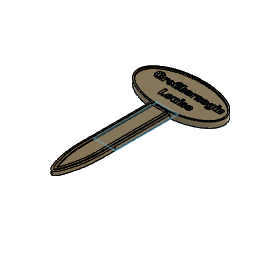
Rosen-Tafel_Großherzoging_Louise v2 (Autodesk Fusion 360 design; units mm, degrees)
Autodesk Fusion 360 part; units mm, degrees
(part 1 of 2)
sketch "Skizze1" plane through (0, 0, 0) normal (0, 0, 1) x (1, 0, 0) in component "Tafe"
  ellipse E0 centre (0, 0) end of major axis (60, 0) minor radius 30
  line L0 (-60, 0) -> (60, 0)
  line L1 (0, -30) -> (0, 30)
  dimension "d1" = 60
  constraint coincident E0.centre origin
  constraint horizontal L0
  constraint coincident E0 L0.start
  constraint coincident E0 L0.end
  constraint coincident E0 L1.start
  constraint coincident E0 L1.end
  measures "d1" distance of E0
extrude "Extrusion1" add sketch "Skizze1" along normal blind 3 makes body 1 in component "Tafe"
sketch "Skizze2" plane through (0, 0, 3) normal (0, 0, 1) x (-1, 0, 0) in component "Tafe"
  ellipse E0 centre (0, 0) end of major axis (-60, 0) minor radius 30
  spline S0 degree 3 poles (61.9509, 0) (61.9509, 4.2635) (60.3055, 8.4828) (57.3091, 12.2636) (52.6449, 18.1488) (44.7166, 23.0684) (34.8255, 26.4973) (25.2136, 29.8294) (13.7584, 31.7256) (2.1658, 31.9316) (-9.8896, 32.1459) (-22.0459, 30.5274) (-32.3487, 27.3124) (-41.3637, 24.4992) (-48.9522, 20.4892) (-54.1681, 15.6411) (-58.1005, 11.9859) (-60.7028, 7.8251) (-61.5993, 3.4465) (-62.4053, -0.4903) (-61.7899, -4.5541) (-59.8722, -8.3093) (-56.3973, -15.1137) (-48.7697, -20.9418) (-38.5998, -25.0786) (-29.6788, -28.7075) (-18.796, -31.0188) (-7.5068, -31.7189) (4.0223, -32.434) (15.9353, -31.462) (26.4461, -28.9362) (36.7725, -26.4548) (45.7187, -22.4959) (52.0049, -17.4981) (56.4978, -13.926) (59.6597, -9.8063) (61.0885, -5.3839) (61.6588, -3.6187) (61.9509, -1.8099) (61.9509, 0) knots -3.141593 -3.141593 -3.141593 -3.141593 -2.764311 -2.764311 -2.764311 -2.177028 -2.177028 -2.177028 -1.606323 -1.606323 -1.606323 -1.012833 -1.012833 -1.012833 -0.49353 -0.49353 -0.49353 -0.102016 -0.102016 -0.102016 0.249996 0.249996 0.249996 0.887852 0.887852 0.887852 1.447382 1.447382 1.447382 2.018805 2.018805 2.018805 2.580199 2.580199 2.580199 2.981436 2.981436 2.981436 3.141593 3.141593 3.141593 3.141593
  dimension "d4" = 1.9509
extrude "Extrusion2" add sketch "Skizze2" along normal blind 2 and the other way blind 2 bodies 1 in component "Tafe"
sketch "Skizze3" plane through (0, 0, 0) normal (0, 0, 1) x (1, 0, 0) in component "Tafe"
extrude "Extrusion3" add 1 faces at (23.0091, -28.1834, 1) along direction (0, 0, -1) blind 1 on bodies 1 bodies 1 in component "Tafe"
sketch "Skizze1 (2)" plane through (0, 0, 0) normal (0, 0, 1) x (1, 0, 0) in component "Ständer"
extrude "Extrusion4" add 2 faces at (23.0091, -28.1834, 0) (8.4972, -9.7981, 0) along direction (0, 0, -1) blind 3 on bodies 1 bodies 1 in component "Tafe"
sketch "Skizze2 (2)" plane through (0, 0, -3) normal (0, 0, -1) x (1, 0, 0) in component "Ständer"
  spline S0 degree 3 poles (-61.9509, 0) (-61.9509, -1.8099) (-61.6588, -3.6187) (-61.0885, -5.3839) (-59.6597, -9.8063) (-56.4978, -13.926) (-52.0049, -17.4981) (-45.7187, -22.4959) (-36.7725, -26.4548) (-26.4461, -28.9362) (-15.9353, -31.462) (-4.0223, -32.434) (7.5068, -31.7189) (18.796, -31.0188) (29.6788, -28.7075) (38.5998, -25.0786) (48.7697, -20.9418) (56.3973, -15.1137) (59.8722, -8.3093) (61.7899, -4.5541) (62.4053, -0.4903) (61.5993, 3.4465) (60.7028, 7.8251) (58.1005, 11.9859) (54.1681, 15.6411) (48.9522, 20.4892) (41.3637, 24.4992) (32.3487, 27.3124) (22.0459, 30.5274) (9.8896, 32.1459) (-2.1658, 31.9316) (-13.7584, 31.7256) (-25.2136, 29.8294) (-34.8255, 26.4973) (-44.7166, 23.0684) (-52.6449, 18.1488) (-57.3091, 12.2636) (-60.3055, 8.4828) (-61.9509, 4.2635) (-61.9509, 0) knots -3.141593 -3.141593 -3.141593 -3.141593 -2.981436 -2.981436 -2.981436 -2.580199 -2.580199 -2.580199 -2.018805 -2.018805 -2.018805 -1.447382 -1.447382 -1.447382 -0.887852 -0.887852 -0.887852 -0.249996 -0.249996 -0.249996 0.102016 0.102016 0.102016 0.49353 0.49353 0.49353 1.012833 1.012833 1.012833 1.606323 1.606323 1.606323 2.177028 2.177028 2.177028 2.764311 2.764311 2.764311 3.141593 3.141593 3.141593 3.141593
  line L0 (15, 20) -> (-15, 20)
  line L1 (-15, 20) -> (-15, 110)
  line L2 (-15, 110) -> (15, 110)
  line L3 (15, 110) -> (15, 20)
  constraint horizontal L0
  constraint vertical L1
  constraint horizontal L2
  constraint vertical L3
extrude "Extrusion1'" add sketch "Skizze2 (2)" against normal blind 5 separate body contours S0 L0 L1 L3 picked at (1.6815, 23.9477) makes body 2 in component "Ständer"
extrude "Extrusion2'" add sketch "Skizze2 (2)" against normal blind 5 contours S0 L1 L2 L3 bodies 2 in component "Ständer"
sketch "Skizze3 (2)" plane through (0, 0, 2) normal (0, 0, 1) x (-1, 0, 0) in component "Ständer"
  line L0 (15, 20) -> (15, 110)
  line L1 (15, 110) -> (-15, 110)
  line L2 (-15, 110) -> (-15, 20)
  line L3 (-15, 20) -> (15, 20)
  spline S0 degree 5 poles (15, 110) (15.0176, 110.8619) (15.0503, 112.5708) (15.0915, 115.0899) (15.1309, 118.3598) (15.1537, 122.2987) (15.1484, 126.0898) (15.1122, 129.7366) (15.0406, 133.2467) (14.9275, 136.6331) (14.7639, 139.9163) (14.5397, 143.1226) (14.2439, 146.2818) (13.867, 149.4242) (13.4012, 152.5784) (12.8426, 155.769) (12.1915, 159.0132) (11.4507, 162.3163) (10.6251, 165.6668) (9.72, 169.0317) (8.7408, 172.3517) (7.6913, 175.5347) (6.574, 178.4677) (5.3908, 181.0335) (4.1426, 183.1253) (2.8302, 184.6621) (1.7296, 185.4171) (0.8758, 185.7125) (0.294, 185.7893) (0, 185.7977) knots 0 0 0 0 0 0 0.04 0.08 0.12 0.16 0.2 0.24 0.28 0.32 0.36 0.4 0.44 0.48 0.52 0.56 0.6 0.64 0.68 0.72 0.76 0.8 0.84 0.88 0.92 0.96 1 1 1 1 1 1
  line L4 (0, -2.5) -> (0, -20)
  spline S1 degree 5 poles (-15, 110) (-15.0176, 110.8619) (-15.0503, 112.5708) (-15.0915, 115.0899) (-15.1309, 118.3598) (-15.1537, 122.2987) (-15.1484, 126.0898) (-15.1122, 129.7366) (-15.0406, 133.2467) (-14.9275, 136.6331) (-14.7639, 139.9163) (-14.5397, 143.1226) (-14.2439, 146.2818) (-13.867, 149.4242) (-13.4012, 152.5784) (-12.8426, 155.769) (-12.1915, 159.0132) (-11.4507, 162.3163) (-10.6251, 165.6668) (-9.72, 169.0317) (-8.7408, 172.3517) (-7.6913, 175.5347) (-6.574, 178.4677) (-5.3908, 181.0335) (-4.1426, 183.1253) (-2.8302, 184.6621) (-1.7296, 185.4171) (-0.8758, 185.7125) (-0.294, 185.7893) (0, 185.7977) knots 0 0 0 0 0 0 0.04 0.08 0.12 0.16 0.2 0.24 0.28 0.32 0.36 0.4 0.44 0.48 0.52 0.56 0.6 0.64 0.68 0.72 0.76 0.8 0.84 0.88 0.92 0.96 1 1 1 1 1 1
  line L5 (14.8117, 100.8471) -> (15.1883, 119.1529)
  line L6 (6.7737, 185.6047) -> (-6.7737, 185.9906)
  line L7 (-14.8117, 100.8471) -> (-15.1883, 119.1529)
  line L8 (-6.7737, 185.6047) -> (6.7737, 185.9906)
  point P0 (15, 134.2579)
  point P1 (13.5579, 151.4378)
  point P2 (9.54, 169.5876)
  point P3 (3.9981, 183.1652)
  point P4 (-15, 134.2579)
  point P5 (-13.5579, 151.4378)
  point P6 (-9.54, 169.5876)
  point P7 (-3.9981, 183.1652)
  constraint coincident L0.end L1.start
  constraint midpoint L0.end L5
  constraint midpoint S0.end L6
  constraint symmetric L0.end L4 L1.end
  constraint symmetric P0 L4 P4
  constraint symmetric P1 L4 P5
  constraint symmetric P2 L4 P6
  constraint symmetric P3 L4 P7
  constraint symmetric S0.end L4 S1.end
  constraint symmetric L4 L5.start L7.start
  constraint symmetric L4 L5.end L7.end
  constraint symmetric L4 L6.start L8.start
  constraint symmetric L4 L6.end L8.end
extrude "Extrusion3'" add sketch "Skizze3 (2)" against normal blind 5 contours L1 S0 S1 bodies 2 in component "Ständer"
sketch "Skizze4" plane through (0, 0, 2) normal (0, 0, 1) x (-1, 0, 0) in component "Ständer"
  line L0 (15, 20) -> (15, 110)
  spline S0 degree 5 poles (15, 110) (15.0176, 110.8619) (15.0503, 112.5708) (15.0915, 115.0899) (15.1309, 118.3598) (15.1537, 122.2987) (15.1484, 126.0898) (15.1122, 129.7366) (15.0406, 133.2467) (14.9275, 136.6331) (14.7639, 139.9163) (14.5397, 143.1226) (14.2439, 146.2818) (13.867, 149.4242) (13.4012, 152.5784) (12.8426, 155.769) (12.1915, 159.0132) (11.4507, 162.3163) (10.6251, 165.6668) (9.72, 169.0317) (8.7408, 172.3517) (7.6913, 175.5347) (6.574, 178.4677) (5.3908, 181.0335) (4.1426, 183.1253) (2.8302, 184.6621) (1.7296, 185.4171) (0.8758, 185.7125) (0.294, 185.7893) (0, 185.7977) knots 0 0 0 0 0 0 0.04 0.08 0.12 0.16 0.2 0.24 0.28 0.32 0.36 0.4 0.44 0.48 0.52 0.56 0.6 0.64 0.68 0.72 0.76 0.8 0.84 0.88 0.92 0.96 1 1 1 1 1 1
  spline S1 degree 5 poles (-15, 110) (-15.0176, 110.8619) (-15.0503, 112.5708) (-15.0915, 115.0899) (-15.1309, 118.3598) (-15.1537, 122.2987) (-15.1484, 126.0898) (-15.1122, 129.7366) (-15.0406, 133.2467) (-14.9275, 136.6331) (-14.7639, 139.9163) (-14.5397, 143.1226) (-14.2439, 146.2818) (-13.867, 149.4242) (-13.4012, 152.5784) (-12.8426, 155.769) (-12.1915, 159.0132) (-11.4507, 162.3163) (-10.6251, 165.6668) (-9.72, 169.0317) (-8.7408, 172.3517) (-7.6913, 175.5347) (-6.574, 178.4677) (-5.3908, 181.0335) (-4.1426, 183.1253) (-2.8302, 184.6621) (-1.7296, 185.4171) (-0.8758, 185.7125) (-0.294, 185.7893) (0, 185.7977) knots 0 0 0 0 0 0 0.04 0.08 0.12 0.16 0.2 0.24 0.28 0.32 0.36 0.4 0.44 0.48 0.52 0.56 0.6 0.64 0.68 0.72 0.76 0.8 0.84 0.88 0.92 0.96 1 1 1 1 1 1
  line L1 (-15, 110) -> (-15, 20)
  line L2 (-15, 20) -> (15, 20)
  spline S2 degree 3 poles (-11.9777, 110.0309) (-11.9779, 110.0412) (-11.9781, 110.0515) (-11.9783, 110.0618) (-12.1467, 118.2962) (-12.1876, 125.6884) (-12.0304, 132.2915) (-11.8915, 138.1249) (-11.5879, 143.3276) (-10.915, 148.5264) (-10.4464, 152.1476) (-9.7926, 155.8041) (-8.949, 159.6156) (-8.1726, 163.1233) (-7.2391, 166.7794) (-6.1929, 170.2595) (-5.0109, 174.1918) (-3.6533, 177.8638) (-2.3593, 180.1318) (-1.7058, 181.2772) (-1.0734, 182.0403) (-0.6357, 182.4064) (-0.297, 182.6897) (-0.1153, 182.7456) (0, 182.7673) knots -0.000287 -0.000287 -0.000287 -0.000287 0 0 0 0.23016 0.23016 0.23016 0.433487 0.433487 0.433487 0.575116 0.575116 0.575116 0.705456 0.705456 0.705456 0.852728 0.852728 0.852728 0.927106 0.927106 0.927106 0.984664 0.984664 0.984664 0.984664
  spline S3 degree 3 poles (11.9777, 110.0309) (11.9779, 110.0412) (11.9781, 110.0515) (11.9783, 110.0618) (12.1467, 118.2962) (12.1876, 125.6884) (12.0304, 132.2915) (11.8915, 138.1249) (11.5879, 143.3276) (10.915, 148.5264) (10.4464, 152.1476) (9.7926, 155.8041) (8.949, 159.6156) (8.1726, 163.1233) (7.2391, 166.7794) (6.1929, 170.2595) (5.0109, 174.1918) (3.6533, 177.8638) (2.3593, 180.1318) (1.7058, 181.2772) (1.0734, 182.0403) (0.6357, 182.4064) (0.297, 182.6897) (0.1153, 182.7456) (0, 182.7673) knots -0.000287 -0.000287 -0.000287 -0.000287 0 0 0 0.23016 0.23016 0.23016 0.433487 0.433487 0.433487 0.575116 0.575116 0.575116 0.705456 0.705456 0.705456 0.852728 0.852728 0.852728 0.927106 0.927106 0.927106 0.984664 0.984664 0.984664 0.984664
  line L3 (11.9777, 23.0223) -> (11.9777, 110.0309)
  line L4 (-11.9777, 23.0223) -> (11.9777, 23.0223)
  line L5 (-11.9777, 110.0309) -> (-11.9777, 23.0223)
  spline S4 degree 3 poles (-9, 110.0613) (-9.0004, 110.0818) (-9.0008, 110.1022) (-9.0013, 110.1226) (-9.1708, 118.4153) (-9.2103, 125.8461) (-9.0484, 132.4316) (-8.9146, 137.8751) (-8.6346, 142.7164) (-8.0427, 147.5055) (-7.6174, 150.9474) (-7.0241, 154.4041) (-6.2475, 158.0272) (-5.5493, 161.2843) (-4.705, 164.6878) (-3.7598, 167.9778) (-2.8347, 171.1978) (-1.801, 174.2968) (-0.8034, 176.5706) (-0.5276, 177.1992) (-0.2561, 177.763) (0, 178.2439) knots -0.000569 -0.000569 -0.000569 -0.000569 0 0 0 0.232641 0.232641 0.232641 0.424939 0.424939 0.424939 0.56314 0.56314 0.56314 0.687378 0.687378 0.687378 0.80897 0.80897 0.80897 0.842587 0.842587 0.842587 0.842587
  spline S5 degree 3 poles (9, 110.0613) (9.0004, 110.0818) (9.0008, 110.1022) (9.0013, 110.1226) (9.1708, 118.4153) (9.2103, 125.8461) (9.0484, 132.4316) (8.9146, 137.8751) (8.6346, 142.7164) (8.0427, 147.5055) (7.6174, 150.9474) (7.0241, 154.4041) (6.2475, 158.0272) (5.5493, 161.2843) (4.705, 164.6878) (3.7598, 167.9778) (2.8347, 171.1978) (1.801, 174.2968) (0.8034, 176.5706) (0.5276, 177.1992) (0.2561, 177.763) (0, 178.2439) knots -0.000569 -0.000569 -0.000569 -0.000569 0 0 0 0.232641 0.232641 0.232641 0.424939 0.424939 0.424939 0.56314 0.56314 0.56314 0.687378 0.687378 0.687378 0.80897 0.80897 0.80897 0.842587 0.842587 0.842587 0.842587
  line L6 (9, 26) -> (9, 110.0613)
  line L7 (-9, 26) -> (9, 26)
  line L8 (-9, 110.0613) -> (-9, 26)
  dimension "d19" = -3.0223
  dimension "d20" = -6
extrude "Extrusion4'" add sketch "Skizze4" along normal blind 1 contours S2 S3 L3 L4 L5 bodies 2 in component "Ständer"
combine "Kombinieren1" operation add target body 1 tool bodies 2 in component "Tafe"
sketch "Skizze1 (3)" plane through (0, 0, 3) normal (0, 0, 1) x (-1, 0, 0)
  ellipse E0 centre (0, 0) end of major axis (-60, 0) minor radius 30
  spline S0 degree 2 poles (40.3376, -15.9435) (39.0443, -15.8724) (37.9926, -15.3181) knots 0 0 0 1 1 1
  spline S1 degree 2 poles (37.9926, -15.3181) (36.9409, -14.7639) (36.2161, -13.8401) knots 0 0 0 1 1 1
  line L0 (36.2161, -13.8401) -> (38.6748, -11.9215)
  spline S2 degree 2 poles (38.6748, -11.9215) (38.9732, -12.3336) (39.4067, -12.5966) knots 0 0 0 1 1 1
  spline S3 degree 2 poles (39.4067, -12.5966) (39.8402, -12.8595) (40.3376, -12.9305) knots 0 0 0 1 1 1
  line L1 (40.3376, -12.9305) -> (40.3376, -15.9435)
  spline S4 degree 2 poles (41.5882, -4.5455) (42.6967, -4.6734) (43.6063, -5.1282) knots 0 0 0 1 1 1
  spline S5 degree 2 poles (43.6063, -5.1282) (44.5159, -5.583) (45.1696, -6.3149) knots 0 0 0 1 1 1
  spline S6 degree 2 poles (45.1696, -6.3149) (45.8234, -7.0468) (46.1787, -8.0203) knots 0 0 0 1 1 1
  spline S7 degree 2 poles (46.1787, -8.0203) (46.534, -8.9938) (46.534, -10.145) knots 0 0 0 1 1 1
  spline S8 degree 2 poles (46.534, -10.145) (46.534, -11.2535) (46.1716, -12.2413) knots 0 0 0 1 1 1
  spline S9 degree 2 poles (46.1716, -12.2413) (45.8092, -13.229) (45.1483, -13.9893) knots 0 0 0 1 1 1
  spline S10 degree 2 poles (45.1483, -13.9893) (44.4874, -14.7497) (43.585, -15.2471) knots 0 0 0 1 1 1
  spline S11 degree 2 poles (43.585, -15.2471) (42.6825, -15.7445) (41.5882, -15.9008) knots 0 0 0 1 1 1
  line L2 (41.5882, -15.9008) -> (41.5882, -12.8168)
  spline S12 degree 2 poles (41.5882, -12.8168) (42.3983, -12.561) (42.9028, -11.8504) knots 0 0 0 1 1 1
  spline S13 degree 2 poles (42.9028, -11.8504) (43.4073, -11.1398) (43.4073, -10.145) knots 0 0 0 1 1 1
  spline S14 degree 2 poles (43.4073, -10.145) (43.4073, -9.6902) (43.2723, -9.2852) knots 0 0 0 1 1 1
  spline S15 degree 2 poles (43.2723, -9.2852) (43.1373, -8.8802) (42.8957, -8.5391) knots 0 0 0 1 1 1
  spline S16 degree 2 poles (42.8957, -8.5391) (42.6541, -8.198) (42.3201, -7.9351) knots 0 0 0 1 1 1
  spline S17 degree 2 poles (42.3201, -7.9351) (41.9862, -7.6721) (41.5882, -7.53) knots 0 0 0 1 1 1
  line L3 (41.5882, -7.53) -> (41.5882, -4.5455)
  line L4 (35.2497, -4.6592) -> (37.751, -4.6592)
  line L5 (37.751, -4.6592) -> (37.751, -5.3982)
  spline S18 degree 2 poles (37.751, -5.3982) (38.3195, -5.0287) (38.9661, -4.7942) knots 0 0 0 1 1 1
  spline S19 degree 2 poles (38.9661, -4.7942) (39.6128, -4.5597) (40.3376, -4.5029) knots 0 0 0 1 1 1
  line L6 (40.3376, -4.5029) -> (40.3376, -7.4021)
  spline S20 degree 2 poles (40.3376, -7.4021) (39.7123, -7.459) (39.3427, -7.6366) knots 0 0 0 1 1 1
  spline S21 degree 2 poles (39.3427, -7.6366) (38.9732, -7.8143) (38.7601, -8.0132) knots 0 0 0 1 1 1
  spline S22 degree 2 poles (38.7601, -8.0132) (38.5185, -8.2406) (38.4048, -8.5106) knots 0 0 0 1 1 1
  line L7 (38.4048, -8.5106) -> (40.0107, -8.5106)
  line L8 (40.0107, -8.5106) -> (40.0107, -10.8698)
  line L9 (40.0107, -10.8698) -> (35.2497, -10.8698)
  line L10 (35.2497, -10.8698) -> (35.2497, -4.6592)
  spline S23 degree 2 poles (28.3854, -9.9318) (28.5133, -9.9318) (28.7123, -9.9247) knots 0 0 0 1 1 1
  spline S24 degree 2 poles (28.7123, -9.9247) (28.9112, -9.9176) (29.1528, -9.8821) knots 0 0 0 1 1 1
  spline S25 degree 2 poles (29.1528, -9.8821) (29.3944, -9.8466) (29.6502, -9.7755) knots 0 0 0 1 1 1
  spline S26 degree 2 poles (29.6502, -9.7755) (29.9061, -9.7044) (30.1334, -9.5623) knots 0 0 0 1 1 1
  line L11 (30.1334, -9.5623) -> (30.1334, -12.0068)
  spline S27 degree 2 poles (30.1334, -12.0068) (29.835, -12.1631) (29.4086, -12.2697) knots 0 0 0 1 1 1
  spline S28 degree 2 poles (29.4086, -12.2697) (28.9823, -12.3763) (28.3854, -12.3763) knots 0 0 0 1 1 1
  line L12 (28.3854, -12.3763) -> (28.3854, -9.9318)
  line L13 (31.3415, -4.6592) -> (34.1696, -4.6592)
  line L14 (34.1696, -4.6592) -> (34.1696, -12.2057)
  line L15 (34.1696, -12.2057) -> (31.3415, -12.2057)
  line L16 (31.3415, -12.2057) -> (31.3415, -4.6592)
  spline S29 degree 2 poles (24.534, -9.6618) (24.875, -9.4913) (25.0882, -9.1573) knots 0 0 0 1 1 1
  spline S30 degree 2 poles (25.0882, -9.1573) (25.3014, -8.8233) (25.3014, -8.4112) knots 0 0 0 1 1 1
  spline S31 degree 2 poles (25.3014, -8.4112) (25.3014, -8.0274) (25.0882, -7.6935) knots 0 0 0 1 1 1
  spline S32 degree 2 poles (25.0882, -7.6935) (24.875, -7.3595) (24.534, -7.1889) knots 0 0 0 1 1 1
  line L17 (24.534, -7.1889) -> (24.534, -4.5171)
  spline S33 degree 2 poles (24.534, -4.5171) (25.344, -4.6166) (25.9978, -4.9577) knots 0 0 0 1 1 1
  spline S34 degree 2 poles (25.9978, -4.9577) (26.6515, -5.2988) (27.0992, -5.8175) knots 0 0 0 1 1 1
  spline S35 degree 2 poles (27.0992, -5.8175) (27.5469, -6.3362) (27.7885, -7.0042) knots 0 0 0 1 1 1
  spline S36 degree 2 poles (27.7885, -7.0042) (28.0301, -7.6721) (28.0301, -8.4112) knots 0 0 0 1 1 1
  spline S37 degree 2 poles (28.0301, -8.4112) (28.0301, -9.1644) (27.7885, -9.8395) knots 0 0 0 1 1 1
  spline S38 degree 2 poles (27.7885, -9.8395) (27.5469, -10.5145) (27.0921, -11.0333) knots 0 0 0 1 1 1
  spline S39 degree 2 poles (27.0921, -11.0333) (26.6373, -11.552) (25.9907, -11.8931) knots 0 0 0 1 1 1
  spline S40 degree 2 poles (25.9907, -11.8931) (25.344, -12.2342) (24.534, -12.3336) knots 0 0 0 1 1 1
  line L18 (24.534, -12.3336) -> (24.534, -9.6618)
  spline S41 degree 2 poles (22.5301, -8.4112) (22.5301, -8.8233) (22.7362, -9.1573) knots 0 0 0 1 1 1
  spline S42 degree 2 poles (22.7362, -9.1573) (22.9422, -9.4913) (23.2975, -9.6618) knots 0 0 0 1 1 1
  line L19 (23.2975, -9.6618) -> (23.2975, -12.3336)
  spline S43 degree 2 poles (23.2975, -12.3336) (22.4874, -12.2342) (21.8408, -11.886) knots 0 0 0 1 1 1
  spline S44 degree 2 poles (21.8408, -11.886) (21.1942, -11.5378) (20.7394, -11.0119) knots 0 0 0 1 1 1
  spline S45 degree 2 poles (20.7394, -11.0119) (20.2846, -10.4861) (20.043, -9.8181) knots 0 0 0 1 1 1
  spline S46 degree 2 poles (20.043, -9.8181) (19.8014, -9.1502) (19.8014, -8.4112) knots 0 0 0 1 1 1
  spline S47 degree 2 poles (19.8014, -8.4112) (19.8014, -7.6864) (20.0359, -7.0184) knots 0 0 0 1 1 1
  spline S48 degree 2 poles (20.0359, -7.0184) (20.2704, -6.3504) (20.7181, -5.8317) knots 0 0 0 1 1 1
  spline S49 degree 2 poles (20.7181, -5.8317) (21.1657, -5.313) (21.8195, -4.9648) knots 0 0 0 1 1 1
  spline S50 degree 2 poles (21.8195, -4.9648) (22.4732, -4.6166) (23.2975, -4.5171) knots 0 0 0 1 1 1
  line L20 (23.2975, -4.5171) -> (23.2975, -7.1889)
  spline S51 degree 2 poles (23.2975, -7.1889) (22.9564, -7.3595) (22.7433, -7.6935) knots 0 0 0 1 1 1
  spline S52 degree 2 poles (22.7433, -7.6935) (22.5301, -8.0274) (22.5301, -8.4112) knots 0 0 0 1 1 1
  spline S53 degree 2 poles (14.8699, -15.9577) (14.1166, -15.9577) (13.4842, -15.7729) knots 0 0 0 1 1 1
  spline S54 degree 2 poles (13.4842, -15.7729) (12.8518, -15.5882) (12.3899, -15.2471) knots 0 0 0 1 1 1
  spline S55 degree 2 poles (12.3899, -15.2471) (11.928, -14.906) (11.6722, -14.4157) knots 0 0 0 1 1 1
  spline S56 degree 2 poles (11.6722, -14.4157) (11.4164, -13.9254) (11.4164, -13.2858) knots 0 0 0 1 1 1
  spline S57 degree 2 poles (11.4164, -13.2858) (11.4164, -12.7174) (11.5798, -12.3123) knots 0 0 0 1 1 1
  spline S58 degree 2 poles (11.5798, -12.3123) (11.7433, -11.9073) (11.9635, -11.6373) knots 0 0 0 1 1 1
  spline S59 degree 2 poles (11.9635, -11.6373) (12.1838, -11.3672) (12.4112, -11.2038) knots 0 0 0 1 1 1
  spline S60 degree 2 poles (12.4112, -11.2038) (12.6386, -11.0404) (12.7807, -10.9693) knots 0 0 0 1 1 1
  spline S61 degree 2 poles (12.7807, -10.9693) (12.4823, -10.8698) (12.0915, -10.6495) knots 0 0 0 1 1 1
  spline S62 degree 2 poles (12.0915, -10.6495) (11.7006, -10.4292) (11.3524, -10.0313) knots 0 0 0 1 1 1
  spline S63 degree 2 poles (11.3524, -10.0313) (11.0042, -9.6334) (10.7697, -9.0294) knots 0 0 0 1 1 1
  spline S64 degree 2 poles (10.7697, -9.0294) (10.5352, -8.4254) (10.5352, -7.5584) knots 0 0 0 1 1 1
  spline S65 degree 2 poles (10.5352, -7.5584) (10.5352, -6.8905) (10.7342, -6.3078) knots 0 0 0 1 1 1
  spline S66 degree 2 poles (10.7342, -6.3078) (10.9332, -5.7251) (11.2956, -5.2917) knots 0 0 0 1 1 1
  spline S67 degree 2 poles (11.2956, -5.2917) (11.658, -4.8582) (12.1696, -4.6095) knots 0 0 0 1 1 1
  spline S68 degree 2 poles (12.1696, -4.6095) (12.6812, -4.3608) (13.3208, -4.3608) knots 0 0 0 1 1 1
  spline S69 degree 2 poles (13.3208, -4.3608) (13.7329, -4.3608) (14.1664, -4.4532) knots 0 0 0 1 1 1
  spline S70 degree 2 poles (14.1664, -4.4532) (14.5998, -4.5455) (14.8699, -4.6308) knots 0 0 0 1 1 1
  line L21 (14.8699, -4.6308) -> (14.4009, -6.9047)
  spline S71 degree 2 poles (14.4009, -6.9047) (14.1593, -6.9047) (13.9532, -7.0468) knots 0 0 0 1 1 1
  spline S72 degree 2 poles (13.9532, -7.0468) (13.7471, -7.1889) (13.5979, -7.395) knots 0 0 0 1 1 1
  spline S73 degree 2 poles (13.5979, -7.395) (13.4487, -7.6011) (13.3705, -7.8427) knots 0 0 0 1 1 1
  spline S74 degree 2 poles (13.3705, -7.8427) (13.2924, -8.0843) (13.2924, -8.2833) knots 0 0 0 1 1 1
  spline S75 degree 2 poles (13.2924, -8.2833) (13.2924, -8.7096) (13.47, -8.9725) knots 0 0 0 1 1 1
  spline S76 degree 2 poles (13.47, -8.9725) (13.6477, -9.2355) (13.8964, -9.3847) knots 0 0 0 1 1 1
  spline S77 degree 2 poles (13.8964, -9.3847) (14.1451, -9.5339) (14.4151, -9.5836) knots 0 0 0 1 1 1
  spline S78 degree 2 poles (14.4151, -9.5836) (14.6851, -9.6334) (14.8557, -9.6334) knots 0 0 0 1 1 1
  line L22 (14.8557, -9.6334) -> (14.8557, -11.9215)
  spline S79 degree 2 poles (14.8557, -11.9215) (14.742, -11.9357) (14.5998, -11.9855) knots 0 0 0 1 1 1
  spline S80 degree 2 poles (14.5998, -11.9855) (14.4577, -12.0352) (14.3298, -12.1347) knots 0 0 0 1 1 1
  spline S81 degree 2 poles (14.3298, -12.1347) (14.2019, -12.2342) (14.1166, -12.3976) knots 0 0 0 1 1 1
  spline S82 degree 2 poles (14.1166, -12.3976) (14.0314, -12.561) (14.0314, -12.8168) knots 0 0 0 1 1 1
  spline S83 degree 2 poles (14.0314, -12.8168) (14.0314, -13.229) (14.2588, -13.4493) knots 0 0 0 1 1 1
  spline S84 degree 2 poles (14.2588, -13.4493) (14.4862, -13.6696) (14.8699, -13.698) knots 0 0 0 1 1 1
  line L23 (14.8699, -13.698) -> (14.8699, -15.9577)
  spline S85 degree 2 poles (18.9345, -12.1063) (18.9345, -12.7032) (18.8492, -13.3143) knots 0 0 0 1 1 1
  spline S86 degree 2 poles (18.8492, -13.3143) (18.7639, -13.9254) (18.4726, -14.4512) knots 0 0 0 1 1 1
  spline S87 degree 2 poles (18.4726, -14.4512) (18.1812, -14.9771) (17.6199, -15.3608) knots 0 0 0 1 1 1
  spline S88 degree 2 poles (17.6199, -15.3608) (17.0585, -15.7445) (16.1063, -15.8866) knots 0 0 0 1 1 1
  line L24 (16.1063, -15.8866) -> (16.1063, -4.6592)
  line L25 (16.1063, -4.6592) -> (18.9345, -4.6592)
  line L26 (18.9345, -4.6592) -> (18.9345, -12.1063)
  spline S89 degree 2 poles (5.7743, -12.1631) (5.5185, -12.2626) (5.2129, -12.3194) knots 0 0 0 1 1 1
  spline S90 degree 2 poles (5.2129, -12.3194) (4.9073, -12.3763) (4.552, -12.3763) knots 0 0 0 1 1 1
  spline S91 degree 2 poles (4.552, -12.3763) (3.8841, -12.3763) (3.4719, -12.1702) knots 0 0 0 1 1 1
  spline S92 degree 2 poles (3.4719, -12.1702) (3.0598, -11.9641) (2.8324, -11.6373) knots 0 0 0 1 1 1
  spline S93 degree 2 poles (2.8324, -11.6373) (2.605, -11.3104) (2.5269, -10.9053) knots 0 0 0 1 1 1
  spline S94 degree 2 poles (2.5269, -10.9053) (2.4487, -10.5003) (2.4487, -10.1166) knots 0 0 0 1 1 1
  line L27 (2.4487, -10.1166) -> (2.4487, -4.6592)
  line L28 (2.4487, -4.6592) -> (5.2769, -4.6592)
  line L29 (5.2769, -4.6592) -> (5.2769, -8.8517)
  spline S95 degree 2 poles (5.2769, -8.8517) (5.2769, -9.2212) (5.3621, -9.5552) knots 0 0 0 1 1 1
  spline S96 degree 2 poles (5.3621, -9.5552) (5.4474, -9.8892) (5.7743, -10.0313) knots 0 0 0 1 1 1
  line L30 (5.7743, -10.0313) -> (5.7743, -12.1631)
  line L31 (7.0107, -4.6592) -> (9.8389, -4.6592)
  line L32 (9.8389, -4.6592) -> (9.8389, -15.6592)
  line L33 (9.8389, -15.6592) -> (7.0107, -15.6592)
  line L34 (7.0107, -15.6592) -> (7.0107, -4.6592)
  line L35 (-1.8149, -9.0649) -> (-3.2787, -9.0649)
  spline S97 degree 2 poles (-3.2787, -9.0649) (-3.2787, -9.3776) (-3.1366, -9.6902) knots 0 0 0 1 1 1
  spline S98 degree 2 poles (-3.1366, -9.6902) (-2.9945, -10.0029) (-2.6534, -10.1592) knots 0 0 0 1 1 1
  line L36 (-2.6534, -10.1592) -> (-2.6534, -12.3479)
  spline S99 degree 2 poles (-2.6534, -12.3479) (-3.4208, -12.2626) (-4.039, -11.9428) knots 0 0 0 1 1 1
  spline S100 degree 2 poles (-4.039, -11.9428) (-4.6573, -11.623) (-5.0907, -11.1043) knots 0 0 0 1 1 1
  spline S101 degree 2 poles (-5.0907, -11.1043) (-5.5242, -10.5856) (-5.7587, -9.8821) knots 0 0 0 1 1 1
  spline S102 degree 2 poles (-5.7587, -9.8821) (-5.9932, -9.1786) (-5.9932, -8.3259) knots 0 0 0 1 1 1
  spline S103 degree 2 poles (-5.9932, -8.3259) (-5.9932, -8.1411) (-5.9221, -7.9706) knots 0 0 0 1 1 1
  line L37 (-5.9221, -7.9706) -> (-1.8149, -7.9706)
  line L38 (-1.8149, -7.9706) -> (-1.8149, -9.0649)
  spline S104 degree 2 poles (-1.4169, -10.1308) (-1.0901, -9.9176) (-0.9337, -9.4842) knots 0 0 0 1 1 1
  spline S105 degree 2 poles (-0.9337, -9.4842) (-0.7774, -9.0507) (-0.7774, -8.5817) knots 0 0 0 1 1 1
  spline S106 degree 2 poles (-0.7774, -8.5817) (-0.7774, -8.0843) (-0.9408, -7.6224) knots 0 0 0 1 1 1
  spline S107 degree 2 poles (-0.9408, -7.6224) (-1.1043, -7.1605) (-1.4169, -6.9615) knots 0 0 0 1 1 1
  line L39 (-1.4169, -6.9615) -> (-1.4169, -4.5313)
  spline S108 degree 2 poles (-1.4169, -4.5313) (-0.6211, -4.6308) (-0.0029, -4.9648) knots 0 0 0 1 1 1
  spline S109 degree 2 poles (-0.0029, -4.9648) (0.6154, -5.2988) (1.0417, -5.8104) knots 0 0 0 1 1 1
  spline S110 degree 2 poles (1.0417, -5.8104) (1.4681, -6.322) (1.6955, -6.99) knots 0 0 0 1 1 1
  spline S111 degree 2 poles (1.6955, -6.99) (1.9229, -7.6579) (1.9229, -8.4254) knots 0 0 0 1 1 1
  spline S112 degree 2 poles (1.9229, -8.4254) (1.9229, -9.1928) (1.6884, -9.8608) knots 0 0 0 1 1 1
  spline S113 degree 2 poles (1.6884, -9.8608) (1.4539, -10.5287) (1.0133, -11.0404) knots 0 0 0 1 1 1
  spline S114 degree 2 poles (1.0133, -11.0404) (0.5727, -11.552) (-0.0384, -11.886) knots 0 0 0 1 1 1
  spline S115 degree 2 poles (-0.0384, -11.886) (-0.6495, -12.2199) (-1.4169, -12.3336) knots 0 0 0 1 1 1
  line L40 (-1.4169, -12.3336) -> (-1.4169, -10.1308)
  spline S116 degree 2 poles (-5.7231, -6.2936) (-5.4815, -5.853) (-5.0836, -5.5119) knots 0 0 0 1 1 1
  spline S117 degree 2 poles (-5.0836, -5.5119) (-4.6857, -5.1709) (-4.103, -4.8866) knots 0 0 0 1 1 1
  spline S118 degree 2 poles (-4.103, -4.8866) (-3.5203, -4.6024) (-2.6534, -4.5171) knots 0 0 0 1 1 1
  line L41 (-2.6534, -4.5171) -> (-2.6534, -6.7768)
  spline S119 degree 2 poles (-2.6534, -6.7768) (-2.9376, -6.8336) (-3.1295, -6.9473) knots 0 0 0 1 1 1
  spline S120 degree 2 poles (-3.1295, -6.9473) (-3.3213, -7.061) (-3.4635, -7.1889) knots 0 0 0 1 1 1
  spline S121 degree 2 poles (-3.4635, -7.1889) (-3.6056, -7.3168) (-3.7051, -7.4732) knots 0 0 0 1 1 1
  line L42 (-3.7051, -7.4732) -> (-5.7231, -6.2936)
  spline S122 degree 2 poles (-12.6159, -9.9318) (-12.488, -9.9318) (-12.289, -9.9247) knots 0 0 0 1 1 1
  spline S123 degree 2 poles (-12.289, -9.9247) (-12.0901, -9.9176) (-11.8485, -9.8821) knots 0 0 0 1 1 1
  spline S124 degree 2 poles (-11.8485, -9.8821) (-11.6069, -9.8466) (-11.3511, -9.7755) knots 0 0 0 1 1 1
  spline S125 degree 2 poles (-11.3511, -9.7755) (-11.0952, -9.7044) (-10.8678, -9.5623) knots 0 0 0 1 1 1
  line L43 (-10.8678, -9.5623) -> (-10.8678, -12.0068)
  spline S126 degree 2 poles (-10.8678, -12.0068) (-11.1663, -12.1631) (-11.5927, -12.2697) knots 0 0 0 1 1 1
  spline S127 degree 2 poles (-11.5927, -12.2697) (-12.019, -12.3763) (-12.6159, -12.3763) knots 0 0 0 1 1 1
  line L44 (-12.6159, -12.3763) -> (-12.6159, -9.9318)
  line L45 (-9.6598, -4.6592) -> (-6.8317, -4.6592)
  line L46 (-6.8317, -4.6592) -> (-6.8317, -12.2057)
  line L47 (-6.8317, -12.2057) -> (-9.6598, -12.2057)
  line L48 (-9.6598, -12.2057) -> (-9.6598, -4.6592)
  line L49 (-18.6702, -6.8194) -> (-20.5035, -6.8194)
  line L50 (-20.5035, -6.8194) -> (-20.5035, -4.6592)
  line L51 (-20.5035, -4.6592) -> (-15.7567, -4.6592)
  line L52 (-15.7567, -4.6592) -> (-18.6702, -6.8194)
  line L53 (-15.302, -10.0029) -> (-13.4402, -10.0029)
  line L54 (-13.4402, -10.0029) -> (-13.4402, -12.2057)
  line L55 (-13.4402, -12.2057) -> (-18.4286, -12.2057)
  line L56 (-18.4286, -12.2057) -> (-15.302, -10.0029)
  line L57 (-13.3976, -4.6592) -> (-13.3976, -7.1889)
  line L58 (-13.3976, -7.1889) -> (-20.5035, -12.2057)
  line L59 (-20.5035, -12.2057) -> (-20.5035, -9.6618)
  line L60 (-20.5035, -9.6618) -> (-13.7387, -4.6592)
  line L61 (-13.7387, -4.6592) -> (-13.3976, -4.6592)
  spline S128 degree 2 poles (-24.5823, -9.6618) (-24.2412, -9.4913) (-24.0281, -9.1573) knots 0 0 0 1 1 1
  spline S129 degree 2 poles (-24.0281, -9.1573) (-23.8149, -8.8233) (-23.8149, -8.4112) knots 0 0 0 1 1 1
  spline S130 degree 2 poles (-23.8149, -8.4112) (-23.8149, -8.0274) (-24.0281, -7.6935) knots 0 0 0 1 1 1
  spline S131 degree 2 poles (-24.0281, -7.6935) (-24.2412, -7.3595) (-24.5823, -7.1889) knots 0 0 0 1 1 1
  line L62 (-24.5823, -7.1889) -> (-24.5823, -4.5171)
  spline S132 degree 2 poles (-24.5823, -4.5171) (-23.7722, -4.6166) (-23.1185, -4.9577) knots 0 0 0 1 1 1
  spline S133 degree 2 poles (-23.1185, -4.9577) (-22.4648, -5.2988) (-22.0171, -5.8175) knots 0 0 0 1 1 1
  spline S134 degree 2 poles (-22.0171, -5.8175) (-21.5694, -6.3362) (-21.3278, -7.0042) knots 0 0 0 1 1 1
  spline S135 degree 2 poles (-21.3278, -7.0042) (-21.0862, -7.6721) (-21.0862, -8.4112) knots 0 0 0 1 1 1
  spline S136 degree 2 poles (-21.0862, -8.4112) (-21.0862, -9.1644) (-21.3278, -9.8395) knots 0 0 0 1 1 1
  spline S137 degree 2 poles (-21.3278, -9.8395) (-21.5694, -10.5145) (-22.0242, -11.0333) knots 0 0 0 1 1 1
  spline S138 degree 2 poles (-22.0242, -11.0333) (-22.479, -11.552) (-23.1256, -11.8931) knots 0 0 0 1 1 1
  spline S139 degree 2 poles (-23.1256, -11.8931) (-23.7722, -12.2342) (-24.5823, -12.3336) knots 0 0 0 1 1 1
  line L63 (-24.5823, -12.3336) -> (-24.5823, -9.6618)
  spline S140 degree 2 poles (-26.5862, -8.4112) (-26.5862, -8.8233) (-26.3801, -9.1573) knots 0 0 0 1 1 1
  spline S141 degree 2 poles (-26.3801, -9.1573) (-26.1741, -9.4913) (-25.8188, -9.6618) knots 0 0 0 1 1 1
  line L64 (-25.8188, -9.6618) -> (-25.8188, -12.3336)
  spline S142 degree 2 poles (-25.8188, -12.3336) (-26.6288, -12.2342) (-27.2755, -11.886) knots 0 0 0 1 1 1
  spline S143 degree 2 poles (-27.2755, -11.886) (-27.9221, -11.5378) (-28.3769, -11.0119) knots 0 0 0 1 1 1
  spline S144 degree 2 poles (-28.3769, -11.0119) (-28.8317, -10.4861) (-29.0733, -9.8181) knots 0 0 0 1 1 1
  spline S145 degree 2 poles (-29.0733, -9.8181) (-29.3149, -9.1502) (-29.3149, -8.4112) knots 0 0 0 1 1 1
  spline S146 degree 2 poles (-29.3149, -8.4112) (-29.3149, -7.6864) (-29.0804, -7.0184) knots 0 0 0 1 1 1
  spline S147 degree 2 poles (-29.0804, -7.0184) (-28.8459, -6.3504) (-28.3982, -5.8317) knots 0 0 0 1 1 1
  spline S148 degree 2 poles (-28.3982, -5.8317) (-27.9505, -5.313) (-27.2968, -4.9648) knots 0 0 0 1 1 1
  spline S149 degree 2 poles (-27.2968, -4.9648) (-26.643, -4.6166) (-25.8188, -4.5171) knots 0 0 0 1 1 1
  line L65 (-25.8188, -4.5171) -> (-25.8188, -7.1889)
  spline S150 degree 2 poles (-25.8188, -7.1889) (-26.1598, -7.3595) (-26.373, -7.6935) knots 0 0 0 1 1 1
  spline S151 degree 2 poles (-26.373, -7.6935) (-26.5862, -8.0274) (-26.5862, -8.4112) knots 0 0 0 1 1 1
  line L66 (-34.5733, -9.8892) -> (-34.2748, -9.9034)
  spline S152 degree 2 poles (-34.2748, -9.9034) (-33.9622, -9.9034) (-33.685, -9.7968) knots 0 0 0 1 1 1
  spline S153 degree 2 poles (-33.685, -9.7968) (-33.4079, -9.6902) (-33.2089, -9.4984) knots 0 0 0 1 1 1
  spline S154 degree 2 poles (-33.2089, -9.4984) (-33.01, -9.3065) (-32.8892, -9.0507) knots 0 0 0 1 1 1
  spline S155 degree 2 poles (-32.8892, -9.0507) (-32.7684, -8.7949) (-32.7684, -8.4964) knots 0 0 0 1 1 1
  spline S156 degree 2 poles (-32.7684, -8.4964) (-32.7684, -7.8285) (-33.2161, -7.4234) knots 0 0 0 1 1 1
  spline S157 degree 2 poles (-33.2161, -7.4234) (-33.6637, -7.0184) (-34.2748, -7.0184) knots 0 0 0 1 1 1
  line L67 (-34.2748, -7.0184) -> (-34.5733, -7.0326)
  line L68 (-34.5733, -7.0326) -> (-34.5733, -4.8156)
  spline S158 degree 2 poles (-34.5733, -4.8156) (-34.3459, -4.7445) (-34.0901, -4.7019) knots 0 0 0 1 1 1
  spline S159 degree 2 poles (-34.0901, -4.7019) (-33.8343, -4.6592) (-33.55, -4.6592) knots 0 0 0 1 1 1
  spline S160 degree 2 poles (-33.55, -4.6592) (-32.7399, -4.6592) (-32.0791, -4.9506) knots 0 0 0 1 1 1
  spline S161 degree 2 poles (-32.0791, -4.9506) (-31.4182, -5.2419) (-30.9564, -5.7535) knots 0 0 0 1 1 1
  spline S162 degree 2 poles (-30.9564, -5.7535) (-30.4945, -6.2652) (-30.2387, -6.9758) knots 0 0 0 1 1 1
  spline S163 degree 2 poles (-30.2387, -6.9758) (-29.9828, -7.6864) (-29.9828, -8.5249) knots 0 0 0 1 1 1
  spline S164 degree 2 poles (-29.9828, -8.5249) (-29.9828, -9.3634) (-30.26, -10.0668) knots 0 0 0 1 1 1
  spline S165 degree 2 poles (-30.26, -10.0668) (-30.5371, -10.7703) (-31.0132, -11.282) knots 0 0 0 1 1 1
  spline S166 degree 2 poles (-31.0132, -11.282) (-31.4893, -11.7936) (-32.1359, -12.0849) knots 0 0 0 1 1 1
  spline S167 degree 2 poles (-32.1359, -12.0849) (-32.7826, -12.3763) (-33.5074, -12.3763) knots 0 0 0 1 1 1
  spline S168 degree 2 poles (-33.5074, -12.3763) (-33.8201, -12.3763) (-34.083, -12.3407) knots 0 0 0 1 1 1
  spline S169 degree 2 poles (-34.083, -12.3407) (-34.3459, -12.3052) (-34.5733, -12.2342) knots 0 0 0 1 1 1
  line L69 (-34.5733, -12.2342) -> (-34.5733, -9.8892)
  line L70 (-35.8097, -12.2057) -> (-38.5952, -12.2057)
  line L71 (-38.5952, -12.2057) -> (-38.5952, -5.782)
  spline S170 degree 2 poles (-38.5952, -5.782) (-38.5952, -4.9861) (-38.4114, -4.1973) knots 0 0 0 1 1 1
  spline S171 degree 2 poles (-38.4114, -4.1973) (-38.2275, -3.4086) (-37.7398, -2.7904) knots 0 0 0 1 1 1
  spline S172 degree 2 poles (-37.7398, -2.7904) (-37.252, -2.1721) (-36.3959, -1.7884) knots 0 0 0 1 1 1
  spline S173 degree 2 poles (-36.3959, -1.7884) (-35.5397, -1.4047) (-34.5733, -1.4047) knots 0 0 0 1 1 1
  spline S174 degree 2 poles (-34.5733, -1.4047) (-33.6069, -1.4047) (-33.0668, -1.5042) knots 0 0 0 1 1 1
  spline S175 degree 2 poles (-33.0668, -1.5042) (-32.5268, -1.6037) (-32.0791, -1.7458) knots 0 0 0 1 1 1
  spline S176 degree 2 poles (-32.0791, -1.7458) (-31.6314, -1.8879) (-31.2832, -2.03) knots 0 0 0 1 1 1
  spline S177 degree 2 poles (-31.2832, -2.03) (-30.935, -2.1721) (-30.7503, -2.2574) knots 0 0 0 1 1 1
  line L72 (-30.7503, -2.2574) -> (-31.6314, -4.176)
  spline S178 degree 2 poles (-31.6314, -4.176) (-31.9157, -3.9913) (-32.2283, -3.8491) knots 0 0 0 1 1 1
  spline S179 degree 2 poles (-32.2283, -3.8491) (-32.541, -3.707) (-32.9105, -3.6075) knots 0 0 0 1 1 1
  spline S180 degree 2 poles (-32.9105, -3.6075) (-33.28, -3.5081) (-34.019, -3.5081) knots 0 0 0 1 1 1
  spline S181 degree 2 poles (-34.019, -3.5081) (-34.758, -3.5081) (-35.2555, -3.8136) knots 0 0 0 1 1 1
  spline S182 degree 2 poles (-35.2555, -3.8136) (-35.7529, -4.1192) (-35.8097, -4.7729) knots 0 0 0 1 1 1
  line L73 (-35.8097, -4.7729) -> (-35.8097, -12.2057)
  line L74 (-39.7038, -12.2057) -> (-42.5319, -12.2057)
  line L75 (-42.5319, -12.2057) -> (-42.5319, -4.6592)
  line L76 (-42.5319, -4.6592) -> (-39.7038, -4.6592)
  line L77 (-39.7038, -4.6592) -> (-39.7038, -12.2057)
  line L78 (-39.7038, -13.2148) -> (-39.7038, -15.645)
  line L79 (-39.7038, -15.645) -> (-42.5319, -15.645)
  line L80 (-42.5319, -15.645) -> (-42.5319, -13.2148)
  line L81 (-42.5319, -13.2148) -> (-39.7038, -13.2148)
  spline S183 degree 2 poles (-47.6766, -12.1063) (-47.9609, -12.2342) (-48.2735, -12.3052) knots 0 0 0 1 1 1
  spline S184 degree 2 poles (-48.2735, -12.3052) (-48.5862, -12.3763) (-48.9557, -12.3763) knots 0 0 0 1 1 1
  spline S185 degree 2 poles (-48.9557, -12.3763) (-50.0216, -12.3763) (-50.519, -11.7794) knots 0 0 0 1 1 1
  spline S186 degree 2 poles (-50.519, -11.7794) (-51.0164, -11.1825) (-51.0164, -10.2729) knots 0 0 0 1 1 1
  line L82 (-51.0164, -10.2729) -> (-51.0164, -4.6592)
  line L83 (-51.0164, -4.6592) -> (-48.1741, -4.6592)
  line L84 (-48.1741, -4.6592) -> (-48.1741, -8.7665)
  spline S187 degree 2 poles (-48.1741, -8.7665) (-48.1741, -8.9228) (-48.1594, -9.1004) knots 0 0 0 1 1 1
  spline S188 degree 2 poles (-48.1594, -9.1004) (-48.1447, -9.2781) (-48.1009, -9.4415) knots 0 0 0 1 1 1
  spline S189 degree 2 poles (-48.1009, -9.4415) (-48.057, -9.605) (-47.9547, -9.7471) knots 0 0 0 1 1 1
  spline S190 degree 2 poles (-47.9547, -9.7471) (-47.8523, -9.8892) (-47.6766, -9.9603) knots 0 0 0 1 1 1
  line L85 (-47.6766, -9.9603) -> (-47.6766, -12.1063)
  line L86 (-43.612, -4.6592) -> (-43.612, -12.2057)
  line L87 (-43.612, -12.2057) -> (-46.4402, -12.2057)
  line L88 (-46.4402, -12.2057) -> (-46.4402, -4.6592)
  line L89 (-46.4402, -4.6592) -> (-43.612, -4.6592)
  line L90 (15.5449, 11.3576) -> (12.063, 11.3576)
  line L91 (12.063, 11.3576) -> (12.063, 13.7878)
  line L92 (12.063, 13.7878) -> (15.5449, 13.7878)
  line L93 (15.5449, 13.7878) -> (15.5449, 11.3576)
  line L94 (19.8938, 13.7878) -> (19.8938, 2.7878)
  line L95 (19.8938, 2.7878) -> (16.7956, 2.7878)
  line L96 (16.7956, 2.7878) -> (16.7956, 13.7878)
  line L97 (16.7956, 13.7878) -> (19.8938, 13.7878)
  spline S191 degree 2 poles (8.3679, 8.7852) (8.709, 8.9558) (8.9222, 9.2897) knots 0 0 0 1 1 1
  spline S192 degree 2 poles (8.9222, 9.2897) (9.1354, 9.6237) (9.1354, 10.0359) knots 0 0 0 1 1 1
  spline S193 degree 2 poles (9.1354, 10.0359) (9.1354, 10.4196) (8.9222, 10.7536) knots 0 0 0 1 1 1
  spline S194 degree 2 poles (8.9222, 10.7536) (8.709, 11.0875) (8.3679, 11.2581) knots 0 0 0 1 1 1
  line L98 (8.3679, 11.2581) -> (8.3679, 13.9299)
  spline S195 degree 2 poles (8.3679, 13.9299) (9.178, 13.8304) (9.8318, 13.4894) knots 0 0 0 1 1 1
  spline S196 degree 2 poles (9.8318, 13.4894) (10.4855, 13.1483) (10.9332, 12.6295) knots 0 0 0 1 1 1
  spline S197 degree 2 poles (10.9332, 12.6295) (11.3809, 12.1108) (11.6225, 11.4428) knots 0 0 0 1 1 1
  spline S198 degree 2 poles (11.6225, 11.4428) (11.8641, 10.7749) (11.8641, 10.0359) knots 0 0 0 1 1 1
  spline S199 degree 2 poles (11.8641, 10.0359) (11.8641, 9.2826) (11.6225, 8.6076) knots 0 0 0 1 1 1
  spline S200 degree 2 poles (11.6225, 8.6076) (11.3809, 7.9325) (10.9261, 7.4138) knots 0 0 0 1 1 1
  spline S201 degree 2 poles (10.9261, 7.4138) (10.4713, 6.895) (9.8247, 6.554) knots 0 0 0 1 1 1
  spline S202 degree 2 poles (9.8247, 6.554) (9.178, 6.2129) (8.3679, 6.1134) knots 0 0 0 1 1 1
  line L99 (8.3679, 6.1134) -> (8.3679, 8.7852)
  spline S203 degree 2 poles (6.3641, 10.0359) (6.3641, 9.6237) (6.5701, 9.2897) knots 0 0 0 1 1 1
  spline S204 degree 2 poles (6.5701, 9.2897) (6.7762, 8.9558) (7.1315, 8.7852) knots 0 0 0 1 1 1
  line L100 (7.1315, 8.7852) -> (7.1315, 6.1134)
  spline S205 degree 2 poles (7.1315, 6.1134) (6.3214, 6.2129) (5.6748, 6.5611) knots 0 0 0 1 1 1
  spline S206 degree 2 poles (5.6748, 6.5611) (5.0281, 6.9093) (4.5734, 7.4351) knots 0 0 0 1 1 1
  spline S207 degree 2 poles (4.5734, 7.4351) (4.1186, 7.9609) (3.877, 8.6289) knots 0 0 0 1 1 1
  spline S208 degree 2 poles (3.877, 8.6289) (3.6354, 9.2968) (3.6354, 10.0359) knots 0 0 0 1 1 1
  spline S209 degree 2 poles (3.6354, 10.0359) (3.6354, 10.7607) (3.8699, 11.4286) knots 0 0 0 1 1 1
  spline S210 degree 2 poles (3.8699, 11.4286) (4.1044, 12.0966) (4.552, 12.6153) knots 0 0 0 1 1 1
  spline S211 degree 2 poles (4.552, 12.6153) (4.9997, 13.1341) (5.6535, 13.4822) knots 0 0 0 1 1 1
  spline S212 degree 2 poles (5.6535, 13.4822) (6.3072, 13.8304) (7.1315, 13.9299) knots 0 0 0 1 1 1
  line L101 (7.1315, 13.9299) -> (7.1315, 11.2581)
  spline S213 degree 2 poles (7.1315, 11.2581) (6.7904, 11.0875) (6.5772, 10.7536) knots 0 0 0 1 1 1
  spline S214 degree 2 poles (6.5772, 10.7536) (6.3641, 10.4196) (6.3641, 10.0359) knots 0 0 0 1 1 1
  line L102 (-1.8504, 6.2413) -> (-4.6359, 6.2413)
  line L103 (-4.6359, 6.2413) -> (-4.6359, 13.7878)
  line L104 (-4.6359, 13.7878) -> (-1.8504, 13.7878)
  line L105 (-1.8504, 13.7878) -> (-1.8504, 6.2413)
  spline S215 degree 2 poles (-0.6566, 13.7025) (-0.3866, 13.8162) (-0.0597, 13.8873) knots 0 0 0 1 1 1
  spline S216 degree 2 poles (-0.0597, 13.8873) (0.2672, 13.9583) (0.6651, 13.9583) knots 0 0 0 1 1 1
  spline S217 degree 2 poles (0.6651, 13.9583) (1.7878, 13.9583) (2.3137, 13.3188) knots 0 0 0 1 1 1
  spline S218 degree 2 poles (2.3137, 13.3188) (2.8395, 12.6793) (2.8395, 11.6418) knots 0 0 0 1 1 1
  line L106 (2.8395, 11.6418) -> (2.8395, 6.2413)
  line L107 (2.8395, 6.2413) -> (-0.0597, 6.2413)
  line L108 (-0.0597, 6.2413) -> (-0.0597, 10.3059)
  spline S219 degree 2 poles (-0.0597, 10.3059) (-0.0597, 11.0307) (-0.1734, 11.2794) knots 0 0 0 1 1 1
  spline S220 degree 2 poles (-0.1734, 11.2794) (-0.2871, 11.5281) (-0.6566, 11.585) knots 0 0 0 1 1 1
  line L109 (-0.6566, 11.585) -> (-0.6566, 13.7025)
  line L110 (-5.7303, 6.2413) -> (-8.5584, 6.2413)
  line L111 (-8.5584, 6.2413) -> (-8.5584, 13.7878)
  line L112 (-8.5584, 13.7878) -> (-5.7303, 13.7878)
  line L113 (-5.7303, 13.7878) -> (-5.7303, 6.2413)
  line L114 (-5.7303, 5.2323) -> (-5.7303, 2.802)
  line L115 (-5.7303, 2.802) -> (-8.5584, 2.802)
  line L116 (-8.5584, 2.802) -> (-8.5584, 5.2323)
  line L117 (-8.5584, 5.2323) -> (-5.7303, 5.2323)
  spline S221 degree 2 poles (-11.7277, 10.8175) (-11.2587, 10.6896) (-10.8607, 10.4835) knots 0 0 0 1 1 1
  spline S222 degree 2 poles (-10.8607, 10.4835) (-10.4628, 10.2775) (-10.1715, 9.9932) knots 0 0 0 1 1 1
  spline S223 degree 2 poles (-10.1715, 9.9932) (-9.8801, 9.709) (-9.7167, 9.3395) knots 0 0 0 1 1 1
  spline S224 degree 2 poles (-9.7167, 9.3395) (-9.5533, 8.97) (-9.5533, 8.501) knots 0 0 0 1 1 1
  spline S225 degree 2 poles (-9.5533, 8.501) (-9.5533, 7.9041) (-9.8091, 7.4351) knots 0 0 0 1 1 1
  spline S226 degree 2 poles (-9.8091, 7.4351) (-10.0649, 6.9661) (-10.5054, 6.6534) knots 0 0 0 1 1 1
  spline S227 degree 2 poles (-10.5054, 6.6534) (-10.946, 6.3408) (-11.5429, 6.1773) knots 0 0 0 1 1 1
  spline S228 degree 2 poles (-11.5429, 6.1773) (-12.1398, 6.0139) (-12.8078, 6.0139) knots 0 0 0 1 1 1
  spline S229 degree 2 poles (-12.8078, 6.0139) (-13.5468, 6.0139) (-14.1721, 6.1631) knots 0 0 0 1 1 1
  spline S230 degree 2 poles (-14.1721, 6.1631) (-14.7974, 6.3124) (-15.2522, 6.4971) knots 0 0 0 1 1 1
  spline S231 degree 2 poles (-15.2522, 6.4971) (-15.7923, 6.7103) (-16.2186, 6.9803) knots 0 0 0 1 1 1
  line L118 (-16.2186, 6.9803) -> (-15.2806, 8.7568)
  spline S232 degree 2 poles (-15.2806, 8.7568) (-14.9822, 8.5578) (-14.6553, 8.4157) knots 0 0 0 1 1 1
  spline S233 degree 2 poles (-14.6553, 8.4157) (-14.3284, 8.2736) (-14.0016, 8.1883) knots 0 0 0 1 1 1
  spline S234 degree 2 poles (-14.0016, 8.1883) (-13.6747, 8.1031) (-13.3905, 8.0604) knots 0 0 0 1 1 1
  spline S235 degree 2 poles (-13.3905, 8.0604) (-13.1062, 8.0178) (-12.893, 8.0178) knots 0 0 0 1 1 1
  spline S236 degree 2 poles (-12.893, 8.0178) (-12.6088, 8.0178) (-12.488, 8.1102) knots 0 0 0 1 1 1
  spline S237 degree 2 poles (-12.488, 8.1102) (-12.3672, 8.2025) (-12.3672, 8.3162) knots 0 0 0 1 1 1
  spline S238 degree 2 poles (-12.3672, 8.3162) (-12.3672, 8.4726) (-12.4951, 8.6147) knots 0 0 0 1 1 1
  spline S239 degree 2 poles (-12.4951, 8.6147) (-12.623, 8.7568) (-12.9215, 8.8705) knots 0 0 0 1 1 1
  line L119 (-12.9215, 8.8705) -> (-11.7277, 10.8175)
  spline S240 degree 2 poles (-13.0352, 14.001) (-11.8556, 14.001) (-10.9602, 13.7096) knots 0 0 0 1 1 1
  spline S241 degree 2 poles (-10.9602, 13.7096) (-10.0649, 13.4183) (-9.1837, 12.7219) knots 0 0 0 1 1 1
  line L120 (-9.1837, 12.7219) -> (-10.2212, 11.0023)
  spline S242 degree 2 poles (-10.2212, 11.0023) (-10.9034, 11.4428) (-11.5784, 11.7271) knots 0 0 0 1 1 1
  spline S243 degree 2 poles (-11.5784, 11.7271) (-12.2535, 12.0113) (-12.7936, 12.0113) knots 0 0 0 1 1 1
  spline S244 degree 2 poles (-12.7936, 12.0113) (-13.1062, 12.0113) (-13.3407, 11.9189) knots 0 0 0 1 1 1
  spline S245 degree 2 poles (-13.3407, 11.9189) (-13.5752, 11.8266) (-13.5752, 11.6276) knots 0 0 0 1 1 1
  spline S246 degree 2 poles (-13.5752, 11.6276) (-13.5752, 11.5281) (-13.4757, 11.4357) knots 0 0 0 1 1 1
  spline S247 degree 2 poles (-13.4757, 11.4357) (-13.3763, 11.3434) (-13.2626, 11.2723) knots 0 0 0 1 1 1
  spline S248 degree 2 poles (-13.2626, 11.2723) (-13.1204, 11.187) (-12.9499, 11.116) knots 0 0 0 1 1 1
  line L121 (-12.9499, 11.116) -> (-14.1721, 9.1547)
  spline S249 degree 2 poles (-14.1721, 9.1547) (-14.5985, 9.2684) (-14.9964, 9.439) knots 0 0 0 1 1 1
  spline S250 degree 2 poles (-14.9964, 9.439) (-15.3943, 9.6095) (-15.6999, 9.8724) knots 0 0 0 1 1 1
  spline S251 degree 2 poles (-15.6999, 9.8724) (-16.0054, 10.1354) (-16.1902, 10.5191) knots 0 0 0 1 1 1
  spline S252 degree 2 poles (-16.1902, 10.5191) (-16.375, 10.9028) (-16.375, 11.4144) knots 0 0 0 1 1 1
  spline S253 degree 2 poles (-16.375, 11.4144) (-16.375, 11.9971) (-16.1405, 12.4732) knots 0 0 0 1 1 1
  spline S254 degree 2 poles (-16.1405, 12.4732) (-15.906, 12.9493) (-15.4725, 13.2904) knots 0 0 0 1 1 1
  spline S255 degree 2 poles (-15.4725, 13.2904) (-15.039, 13.6315) (-14.4208, 13.8162) knots 0 0 0 1 1 1
  spline S256 degree 2 poles (-14.4208, 13.8162) (-13.8026, 14.001) (-13.0352, 14.001) knots 0 0 0 1 1 1
  line L122 (-20.6101, 9.3821) -> (-22.0739, 9.3821)
  spline S257 degree 2 poles (-22.0739, 9.3821) (-22.0739, 9.0695) (-21.9318, 8.7568) knots 0 0 0 1 1 1
  spline S258 degree 2 poles (-21.9318, 8.7568) (-21.7897, 8.4441) (-21.4486, 8.2878) knots 0 0 0 1 1 1
  line L123 (-21.4486, 8.2878) -> (-21.4486, 6.0992)
  spline S259 degree 2 poles (-21.4486, 6.0992) (-22.216, 6.1844) (-22.8343, 6.5042) knots 0 0 0 1 1 1
  spline S260 degree 2 poles (-22.8343, 6.5042) (-23.4525, 6.824) (-23.8859, 7.3427) knots 0 0 0 1 1 1
  spline S261 degree 2 poles (-23.8859, 7.3427) (-24.3194, 7.8615) (-24.5539, 8.5649) knots 0 0 0 1 1 1
  spline S262 degree 2 poles (-24.5539, 8.5649) (-24.7884, 9.2684) (-24.7884, 10.1211) knots 0 0 0 1 1 1
  spline S263 degree 2 poles (-24.7884, 10.1211) (-24.7884, 10.3059) (-24.7173, 10.4764) knots 0 0 0 1 1 1
  line L124 (-24.7173, 10.4764) -> (-20.6101, 10.4764)
  line L125 (-20.6101, 10.4764) -> (-20.6101, 9.3821)
  spline S264 degree 2 poles (-20.2122, 8.3162) (-19.8853, 8.5294) (-19.729, 8.9629) knots 0 0 0 1 1 1
  spline S265 degree 2 poles (-19.729, 8.9629) (-19.5726, 9.3963) (-19.5726, 9.8653) knots 0 0 0 1 1 1
  spline S266 degree 2 poles (-19.5726, 9.8653) (-19.5726, 10.3627) (-19.7361, 10.8246) knots 0 0 0 1 1 1
  spline S267 degree 2 poles (-19.7361, 10.8246) (-19.8995, 11.2865) (-20.2122, 11.4855) knots 0 0 0 1 1 1
  line L126 (-20.2122, 11.4855) -> (-20.2122, 13.9157)
  spline S268 degree 2 poles (-20.2122, 13.9157) (-19.4163, 13.8162) (-18.7981, 13.4822) knots 0 0 0 1 1 1
  spline S269 degree 2 poles (-18.7981, 13.4822) (-18.1799, 13.1483) (-17.7535, 12.6366) knots 0 0 0 1 1 1
  spline S270 degree 2 poles (-17.7535, 12.6366) (-17.3272, 12.125) (-17.0998, 11.4571) knots 0 0 0 1 1 1
  spline S271 degree 2 poles (-17.0998, 11.4571) (-16.8724, 10.7891) (-16.8724, 10.0217) knots 0 0 0 1 1 1
  spline S272 degree 2 poles (-16.8724, 10.0217) (-16.8724, 9.2542) (-17.1069, 8.5863) knots 0 0 0 1 1 1
  spline S273 degree 2 poles (-17.1069, 8.5863) (-17.3414, 7.9183) (-17.7819, 7.4067) knots 0 0 0 1 1 1
  spline S274 degree 2 poles (-17.7819, 7.4067) (-18.2225, 6.895) (-18.8336, 6.5611) knots 0 0 0 1 1 1
  spline S275 degree 2 poles (-18.8336, 6.5611) (-19.4447, 6.2271) (-20.2122, 6.1134) knots 0 0 0 1 1 1
  line L127 (-20.2122, 6.1134) -> (-20.2122, 8.3162)
  spline S276 degree 2 poles (-24.5184, 12.1534) (-24.2768, 12.594) (-23.8788, 12.9351) knots 0 0 0 1 1 1
  spline S277 degree 2 poles (-23.8788, 12.9351) (-23.4809, 13.2762) (-22.8982, 13.5604) knots 0 0 0 1 1 1
  spline S278 degree 2 poles (-22.8982, 13.5604) (-22.3155, 13.8447) (-21.4486, 13.9299) knots 0 0 0 1 1 1
  line L128 (-21.4486, 13.9299) -> (-21.4486, 11.6702)
  spline S279 degree 2 poles (-21.4486, 11.6702) (-21.7328, 11.6134) (-21.9247, 11.4997) knots 0 0 0 1 1 1
  spline S280 degree 2 poles (-21.9247, 11.4997) (-22.1166, 11.386) (-22.2587, 11.2581) knots 0 0 0 1 1 1
  spline S281 degree 2 poles (-22.2587, 11.2581) (-22.4008, 11.1302) (-22.5003, 10.9739) knots 0 0 0 1 1 1
  line L129 (-22.5003, 10.9739) -> (-24.5184, 12.1534)